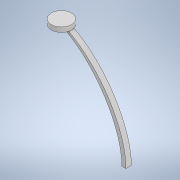
# Autodesk Inventor part: preBuiltArm
Saved by Autodesk Inventor 2020 (Build 240168000, 168)
## iProperties
Created: 2019-06-21
Part Number: preBuiltArm
Material: Generic
Document SubType Name: Modeling
Designer: Vivek Muskan
Density: 1 g/cm^3
Appearance: Default
Author: Vivek Muskan
Autodesk Inventor part; units mm, degrees
ref_plane "YZ Plane" through (0, 0, 0) normal (1, 0, 0) x (0, 1, 0)
ref_plane "XZ Plane" through (0, 0, 0) normal (0, 1, 0) x (-1, 0, 0)
ref_plane "XY Plane" through (0, 0, 0) normal (0, 0, 1) x (1, 0, 0)
sketch "Sketch1" plane through (0, 0, 0) normal (0, 1, 0) x (-1, 0, 0)
  circle A0 centre (0, 0) radius 15
  dimension "d0" = 30
  constraints: 1 centre point, 1 coincident
  measures "d0" diameter of A0
extrude "Extrusion1" add sketch "Sketch1" along normal blind 7
sketch "Sketch2" plane through (0, 0, 0) normal (0, 0, 1) x (1, 0, 0)
  line L0 (0, -0.6683) -> (0, -150.6683)
  line L1 (0, -150.6683) -> (100, -150.6683)
  line L2 (15, 0) -> (-15, 0) projected
  line L3 (15, 0) -> (61.733, -24.0013) construction
  line L4 (61.733, -24.0013) -> (100, -85.3679) construction
  line L5 (100, -85.3679) -> (100, -133.998) construction
  spline S0 degree 3 poles (15, 0) (61.733, -24.0013) (100, -85.3679) (100, -133.998) knots 1 1 1 1 2 2 2 2
  line L6 (8.9554, -0.4801) -> (55.6884, -24.4814) construction
  line L7 (55.6884, -24.4814) -> (93.9554, -85.848) construction
  line L8 (93.9554, -85.848) -> (93.9554, -134.4781) construction
  spline S1 degree 3 poles (8.9554, -0.4801) (55.6884, -24.4814) (93.9554, -85.848) (93.9554, -134.4781) knots 1 1 1 1 2 2 2 2
  line L9 (100, -133.998) -> (93.9542, -133.998)
  line L10 (15, 0) -> (8.9554, 0)
  line L11 (8.9554, -0.4801) -> (8.9554, 0)
  point P0 (0, 0)
  dimension "d3" = 150
  dimension "d4" = 100
  constraints: 10 end point, 2 horizontal, 2 vertical, 1 perpendicular, 1 point on line, 7 other
  measures "d3" distance of L0.start L0.end
  measures "d4" distance of L0.end L1.end
extrude "Extrusion2" add sketch "Sketch2" along normal mid plane 8
body "Solid1"
